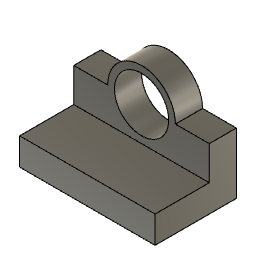
random practice 1 v1 (Autodesk Fusion 360 design; units mm, degrees)
Autodesk Fusion 360 part; units mm, degrees
note: some values were not read from the file. Set by a fixed rule: which sketch regions a step uses; which face or edge a step refers to.
sketch "Sketch1" plane through (0, 0, 0) normal (1, 0, 0) x (0, 1, 0)
  line L0 (0, 0) -> (60, 0)
  line L1 (60, 0) -> (60, 20)
  line L2 (60, 20) -> (0, 20)
  line L3 (0, 20) -> (0, 0)
  line L4 (60, 0) -> (40, 0)
  line L5 (40, 0) -> (40, 45)
  line L6 (40, 45) -> (60, 45)
  line L7 (60, 45) -> (60, 0)
  dimension "d1" = 60
  dimension "d2" = 20
  dimension "d3" = 20
  dimension "d4" = 45
  constraint horizontal L0
  constraint vertical L1
  constraint horizontal L2
  constraint vertical L3
  constraint coincident L0.start L3.end
  constraint horizontal L4
  constraint vertical L5
  constraint horizontal L6
  constraint vertical L7
  measures "d1" distance of L0.start L0.end
  measures "d2" distance of L0.start L2.end
  measures "d3" distance of L0.end L4.end
  measures "d4" distance of L0.end L6.end
extrude "Extrude1" add sketch "Sketch1" along normal blind 100
sketch "Sketch2" plane through (0, 40, 0) normal (0, -1, 0) x (1, 0, 0)
  line L0 (0, 45) -> (0, 20)
  line L1 (0, 20) -> (100, 20)
  line L2 (100, 20) -> (100, 45)
  line L3 (100, 45) -> (0, 45)
  circle A0 centre (50, 45) radius 25
  dimension "d7" = 50
  constraint midpoint L3 A0.centre
  measures "d7" diameter of A0
extrude "Extrude2" add sketch "Sketch2" against normal up to surface (20 mm away) contours L3 A0 picked at (47.8685, 56.8227)
sketch "Sketch3" plane through (0, 40, 0) normal (0, -1, 0) x (1, 0, 0)
  line L0 (0, 45) -> (0, 20)
  line L1 (0, 20) -> (100, 20)
  line L2 (100, 20) -> (100, 45)
  line L3 (100, 45) -> (75, 45)
  arc A0 (75, 45) -> (25, 45) centre (50, 45) ccw
  line L4 (25, 45) -> (0, 45)
  circle A1 centre (50, 45) radius 20
  dimension "d10" = 40
  constraint concentric A0 A1
  measures "d10" diameter of A1
extrude "Extrude3" cut sketch "Sketch3" against normal through all contours A1
